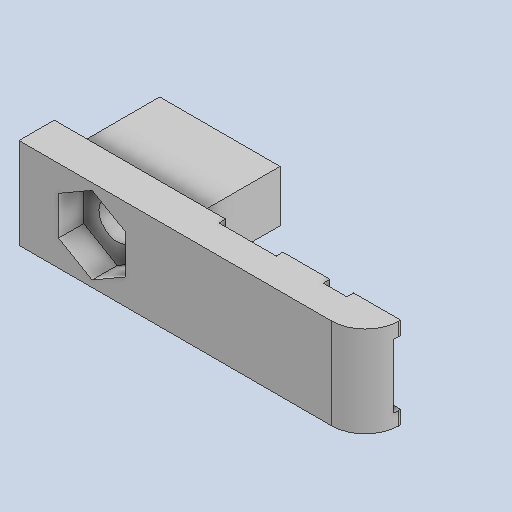
# Autodesk Inventor part: stereotax_holder_side
Saved by Autodesk Inventor 2023.3 (Build 273359000, 359)
## iProperties
Created: 2023-10-03
Part Number: stereotax_holder_side
Material: Generic
Document SubType Name: Modeling
Designer: mmelin
Density: 1 g/cm^3
Appearance: Default
Author: mmelin
Autodesk Inventor part; units mm, degrees
ref_plane "YZ Plane" through (0, 0, 0) normal (1, 0, 0) x (0, 1, 0)
ref_plane "XZ Plane" through (0, 0, 0) normal (0, 1, 0) x (-1, 0, 0)
ref_plane "XY Plane" through (0, 0, 0) normal (0, 0, 1) x (1, 0, 0)
sketch "Sketch1" plane through (0, 0, 0) normal (0, 0, 1) x (1, 0, 0)
  line L0 (-6.6, -4.4) -> (-23.2373, -4.4) projected
  line L1 (-23.2373, 1) -> (-6.6, 1) projected
  line L2 (-4.6, -4.4) -> (-25.2, -4.4)
  line L3 (-25.2, -4.4) -> (-25.2, 1)
  line L4 (-25.2, 1) -> (-4.6, 1)
  line L5 (-4.6, 1) -> (-4.6, -4.4)
  line L6 (-11.6, -0.9) -> (-11.6, -3.4) projected
  point P0 (0, 0)
  dimension "d0" = 7
  dimension "d1" = 20.6
  constraints: 8 end point, 2 collinear, 2 parallel, 1 horizontal, 1 perpendicular
  measures "d0" distance between parallel lines of L6 L5
  measures "d1" distance between parallel lines of L3 L5
extrude "Extrusion1" add sketch "Sketch1" along normal blind 1.7
sketch "Sketch2" plane through (0, 0, 0) normal (0, 0, -1) x (-1, 0, 0)
  line L0 (4.6, 1) -> (7.4, 1) projected
  line L1 (7.4, 1) -> (7.4, 0.2) projected
  line L2 (7.4, 0.2) -> (4.6, 0.2) projected
  line L3 (4.6, 0.2) -> (4.6, 1) projected
  line L4 (8.8, 0.2) -> (8.8, 1) projected
  line L5 (8.8, 1) -> (11.6, 1) projected
  line L6 (11.6, 1) -> (11.6, 0.2) projected
  line L7 (11.6, 0.2) -> (8.8, 0.2) projected
  line L8 (4.6, -3.6) -> (7.4, -3.6) projected
  line L9 (7.4, -3.6) -> (7.4, -4.4) projected
  line L10 (7.4, -4.4) -> (4.6, -4.4) projected
  line L11 (4.6, -4.4) -> (4.6, -3.6) projected
  line L12 (11.6, -3.6) -> (11.6, -4.4) projected
  line L13 (11.6, -4.4) -> (8.8, -4.4) projected
  line L14 (8.8, -4.4) -> (8.8, -3.6) projected
  line L15 (8.8, -3.6) -> (11.6, -3.6) projected
  line L16 (15, 0) -> (15, -0.9) projected
  line L17 (11.6, -4.4) -> (8.8, -4.4)
  line L18 (8.8, -4.4) -> (8.8, -3.6)
  line L19 (8.8, -3.6) -> (11.6, -3.6)
  line L20 (11.6, -3.6) -> (11.6, -4.4)
  line L21 (7.4, -4.4) -> (4.6, -4.4)
  line L22 (4.6, -4.4) -> (4.6, -3.6)
  line L23 (4.6, -3.6) -> (7.4, -3.6)
  line L24 (7.4, -3.6) -> (7.4, -4.4)
  line L25 (4.6, 0.2) -> (7.4, 0.2)
  line L26 (7.4, 0.2) -> (7.4, 1)
  line L27 (7.4, 1) -> (4.6, 1)
  line L28 (4.6, 1) -> (4.6, 0.2)
  line L29 (8.8, 0.2) -> (11.6, 0.2)
  line L30 (11.6, 0.2) -> (11.6, 1)
  line L31 (11.6, 1) -> (8.8, 1)
  line L32 (8.8, 1) -> (8.8, 0.2)
  line L33 (25.2, -4.4) -> (4.6, -4.4) projected
  line L34 (4.6, 1) -> (25.2, 1) projected
  line L35 (15, -4.4) -> (25.2, -4.4)
  line L36 (25.2, -4.4) -> (25.2, 1)
  line L37 (25.2, 1) -> (15, 1)
  line L38 (15, 1) -> (15, -4.4)
  line L39 (25.2, 1) -> (25.2, -4.4) projected
  point P0 (0, 0)
  constraints: 40 end point, 10 parallel, 5 horizontal, 5 perpendicular, 2 collinear, 2 point on line
extrude "Extrusion2" add sketch "Sketch2" along normal blind 0.4
fillet "Fillet1" radius 2 1 edges at (-4.6, -1.7, 1.7)
sketch "Sketch4" plane through (0, 0, -0.4) normal (0, 0, -1) x (-1, 0, 0)
  line L0 (24.43, -3.23) -> (17.27, -3.23)
  line L1 (17.27, -3.23) -> (17.27, -0.17)
  line L2 (17.27, -0.17) -> (24.43, -0.17)
  line L3 (24.43, -0.17) -> (24.43, -3.23)
  line L4 (24.6, -3.4) -> (24.6, 0) projected
  line L5 (17.1, -3.4) -> (24.6, -3.4) projected
  line L6 (17.1, 0) -> (17.1, -3.4) projected
  line L7 (24.6, 0) -> (17.1, 0) projected
  circle A0 centre (20.85, -1.7) radius 1.1 projected
  circle A1 centre (20.85, -1.7) radius 1.1
  point P0 (0, 0)
  dimension "d14" = 0.17
  dimension "d15" = 0.17
  dimension "d16" = 0.17
  dimension "d17" = 0.17
  constraints: 8 end point, 2 parallel, 1 centre point, 1 coincident, 1 concentric, 1 horizontal, 1 perpendicular
  measures "d14" distance between parallel lines of L7 L2
  measures "d15" distance between parallel lines of L6 L1
  measures "d16" distance between parallel lines of L4 L3
  measures "d17" distance between parallel lines of L5 L0
extrude "Extrusion5" add sketch "Sketch4" along normal blind 5.5 contours L0 L1 L2 L3
sketch "Sketch6" plane through (0, 0, 1.7) normal (0, 0, 1) x (1, 0, 0)
  circle A0 centre (-20.85, -1.7) radius 1.1 projected
  circle A1 centre (-20.85, -1.7) radius 1.1
  point P0 (0, 0)
  constraints: 1 centre point, 1 coincident
extrude "Extrusion7" cut sketch "Sketch6" against normal up to surface (7.6 mm away)
sketch "Sketch7" plane through (0, 0, 1.7) normal (0, 0, 1) x (1, 0, 0)
  circle A0 centre (-20.85, -1.7) radius 1.1 projected
  line L0 (-18.85, -2.8547) -> (-20.85, -4.0094)
  line L1 (-20.85, -4.0094) -> (-22.85, -2.8547)
  line L2 (-22.85, -2.8547) -> (-22.85, -0.5453)
  line L3 (-22.85, -0.5453) -> (-20.85, 0.6094)
  line L4 (-20.85, 0.6094) -> (-18.85, -0.5453)
  line L5 (-18.85, -0.5453) -> (-18.85, -2.8547)
  point P0 (0, 0)
  dimension "d27" = 4
  constraints: 12 end point, 1 coincident, 1 vertical, 13 other
  measures "d27" distance between parallel lines of L5 L2
extrude "Extrusion8" cut sketch "Sketch7" against normal blind 1.5
equation "\"d15\" = d14"
equation "\"d16\" = d14"
equation "\"d17\" = d14"
body "Solid1"
